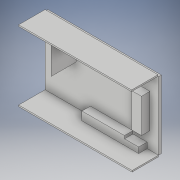
# Autodesk Inventor part: Room3L10
Saved by Autodesk Inventor 2019 (Build 230136000, 136)
## iProperties
Created: 2021-05-11
Part Number: Room3L10
Material: Generic
Document SubType Name: Modeling
Designer: jamieson-bl
Density: 1 g/cm^3
Appearance: Default
Author: jamieson-bl
Autodesk Inventor part; units mm, degrees
ref_plane "YZ Plane" through (0, 0, 0) normal (1, 0, 0) x (0, 1, 0)
ref_plane "XZ Plane" through (0, 0, 0) normal (0, 1, 0) x (-1, 0, 0)
ref_plane "XY Plane" through (0, 0, 0) normal (0, 0, 1) x (1, 0, 0)
sketch "Sketch1" plane through (0, 0, 0) normal (0, 0, 1) x (1, 0, 0)
  line L0 (6096, -3657.6) -> (-6096, -3657.6)
  line L1 (-6096, -3657.6) -> (-6096, 3657.6)
  line L2 (-6096, 3657.6) -> (6096, 3657.6)
  line L3 (6096, 3657.6) -> (6096, -3657.6)
  line L4 (6096, -3657.6) -> (-6096, 3657.6) construction
  line L5 (-6096, -3657.6) -> (6096, 3657.6) construction
  point P0 (0, 0)
  dimension "d0" = 12192
  dimension "d1" = 7315.2
  constraints: 12 end point, 2 midpoint, 2 parallel, 1 horizontal, 1 perpendicular
  measures "d0" distance of L1.end L2.end
  measures "d1" distance of L0.end L1.end
extrude "Floor" add sketch "Sketch1" along normal blind 304.8
sketch "Sketch2" plane through (0, 0, 304.8) normal (0, 0, 1) x (1, 0, 0)
  line L0 (4114.8, 1828.8) -> (5181.6, 1828.8)
  line L1 (5181.6, 1828.8) -> (5181.6, -1828.8)
  line L2 (5181.6, -1828.8) -> (4114.8, -1828.8)
  line L3 (4114.8, -1828.8) -> (4114.8, 1828.8)
  line L4 (4114.8, 1828.8) -> (5181.6, -1828.8) construction
  line L5 (5181.6, 1828.8) -> (4114.8, -1828.8) construction
  line L6 (6096, -3657.6) -> (6096, 3657.6) projected
  line L7 (-6096, -3657.6) -> (6096, -3657.6) projected
  point P0 (0, 0)
  point P1 (4648.2, 0)
  dimension "d4" = 914.4
  dimension "d5" = 1828.8
  dimension "d6" = 1066.8
  dimension "d7" = 3657.6
  constraints: 12 end point, 2 midpoint, 2 parallel, 1 horizontal, 1 perpendicular
  measures "d4" distance between parallel lines of L6 L1
  measures "d5" distance between parallel lines of L7 L2
  measures "d6" distance between parallel lines of L1 L3
  measures "d7" distance of L2.end L0.start
extrude "Desk" add sketch "Sketch2" along normal blind 914.4
sketch "Sketch3" plane through (0, 0, 304.8) normal (0, 0, 1) x (1, 0, 0)
  line L0 (3352.8, -3048) -> (4876.8, -3048)
  line L1 (4876.8, -3048) -> (4876.8, -3657.6)
  line L2 (4876.8, -3657.6) -> (3352.8, -3657.6)
  line L3 (3352.8, -3657.6) -> (3352.8, -3048)
  line L4 (3352.8, -3048) -> (4876.8, -3657.6) construction
  line L5 (4876.8, -3048) -> (3352.8, -3657.6) construction
  line L6 (6096, -3657.6) -> (6096, 3657.6) projected
  line L7 (-6096, -3657.6) -> (6096, -3657.6) projected
  line L8 (-6096, 0) -> (6153.2675, 0) construction
  line L9 (3352.8, 3048) -> (4876.8, 3048)
  line L10 (4876.8, 3048) -> (4876.8, 3657.6)
  line L11 (4876.8, 3657.6) -> (3352.8, 3657.6)
  line L12 (3352.8, 3657.6) -> (3352.8, 3048)
  point P0 (0, 0)
  point P1 (4114.8, -3352.8)
  point P2 (4114.8, 3352.8)
  dimension "d10" = 609.6
  dimension "d11" = 1524
  dimension "d12" = 1219.2
  dimension "d13" = 0
  constraints: 22 end point, 5 symmetric about line, 2 horizontal, 2 midpoint, 2 parallel, 1 perpendicular
  measures "d10" distance of L2.end L0.start
  measures "d11" distance of L0.start L0.end
  measures "d12" distance between parallel lines of L1 L6
  measures "d13" distance between parallel lines of L7 L2
extrude "Sinks" add sketch "Sketch3" along normal blind 914.4
sketch "Sketch4" plane through (0, 0, 304.8) normal (0, 0, 1) x (1, 0, 0)
  line L0 (3352.8, 3657.6) -> (-2743.2, 3657.6)
  line L1 (-2743.2, 3657.6) -> (-2743.2, 2743.2)
  line L2 (-2743.2, 2743.2) -> (3352.8, 2743.2)
  line L3 (3352.8, 2743.2) -> (3352.8, 3657.6)
  line L4 (3352.8, -3657.6) -> (4876.8, -3657.6) projected
  line L5 (3352.8, -3657.6) -> (-1219.2, -3657.6)
  line L6 (-1219.2, -3657.6) -> (-1219.2, -2743.2)
  line L7 (-1219.2, -2743.2) -> (3352.8, -2743.2)
  line L8 (3352.8, -2743.2) -> (3352.8, -3657.6)
  point P0 (0, 0)
  dimension "d16" = 914.4
  dimension "d17" = 6096
  dimension "d18" = 4572
  dimension "d19" = 914.4
  constraints: 16 end point, 4 parallel, 2 horizontal, 2 perpendicular
  measures "d16" distance of L1.end L0.end
  measures "d17" distance of L1.end L2.end
  measures "d18" distance of L6.end L7.end
  measures "d19" distance of L5.end L6.end
extrude "Counters" add sketch "Sketch4" along normal blind 914.4
sketch "Sketch5" plane through (0, 0, 304.8) normal (0, 0, 1) x (1, 0, 0)
  line L0 (-6096, 3657.6) -> (-6096, -3657.6) projected
  line L1 (-6096, 3657.6) -> (6041.772, 3657.6)
  line L2 (6041.772, 3657.6) -> (6041.772, 3810)
  line L3 (6041.772, 3810) -> (-6096, 3810)
  line L4 (-6096, 3810) -> (-6096, 3657.6)
  line L5 (4876.8, -3657.6) -> (6096, -3657.6) projected
  line L6 (6096, -3657.6) -> (-6096, -3657.6)
  line L7 (-6096, -3657.6) -> (-6096, -3810)
  line L8 (-6096, -3810) -> (6096, -3810)
  line L9 (6096, -3810) -> (6096, -3657.6)
  point P0 (0, 0)
  dimension "d22" = 152.4
  dimension "d23" = 152.4
  constraints: 16 end point, 4 parallel, 2 horizontal, 2 perpendicular
  measures "d22" distance of L2.end L1.end
  measures "d23" distance of L7.end L6.end
extrude "Room Walls" add sketch "Sketch5" along normal blind 2844.8
sketch "Sketch6" plane through (-6096, 3657.6, 304.8) normal (0, -1, 0) x (1, 0, 0)
  line L0 (12192, 0) -> (12192, 2844.8) projected
  line L1 (0, 0) -> (0, 2844.8) projected
  line L2 (12192, 2844.8) -> (0, 2844.8)
  line L3 (0, 2844.8) -> (0, 2692.4)
  line L4 (0, 2692.4) -> (12192, 2692.4)
  line L5 (12192, 2692.4) -> (12192, 2844.8)
  point P0 (6096, -304.8)
  dimension "d26" = 152.4
  constraints: 8 end point, 2 parallel, 1 horizontal, 1 perpendicular, 1 point on line
  measures "d26" distance of L3.end L2.end
extrude "Roof" [suppressed]
sketch "Sketch7" plane through (0, 0, 304.8) normal (0, 0, 1) x (1, 0, 0)
  line L0 (-2743.2, 3657.6) -> (-2743.9938, 3657.6)
  line L1 (-2743.9938, 3657.6) -> (-2743.9938, 609.6)
  line L2 (-2743.9938, 609.6) -> (-2743.2, 609.6)
  line L3 (-2743.2, 609.6) -> (-2743.2, 3657.6)
  point P0 (0, 0)
  dimension "d29" = 0.7937
  dimension "d30" = 3048
  constraints: 8 end point, 2 parallel, 1 horizontal, 1 perpendicular
  measures "d29" distance of L2.end L1.end
  measures "d30" distance of L1.end L0.end
extrude "Extrusion7" add sketch "Sketch7" along normal blind 2692.4
body "Solid1"
